# Autodesk Inventor part: finish
Saved by Autodesk Inventor 2022.2 (Build 262287000, 287)
## iProperties
Created: 2021-01-02
Part Number: finish
Material: Generic
Document SubType Name: Modeling
Designer: Tomasz
Density: 1 g/cm^3
Appearance: Default
Author: Tomasz
Autodesk Inventor part; units mm, degrees
ref_plane "YZ Plane" through (0, 0, 0) normal (1, 0, 0) x (0, 1, 0)
ref_plane "XZ Plane" through (0, 0, 0) normal (0, 1, 0) x (-1, 0, 0)
ref_plane "XY Plane" through (0, 0, 0) normal (0, 0, 1) x (1, 0, 0)
sketch "Sketch1" plane through (0, 0, 0) normal (0, 1, 0) x (-1, 0, 0)
  line L0 (275, 0) -> (-275, 0)
  line L1 (-275, 0) -> (-275, -720)
  line L2 (-275, -720) -> (275, -720)
  line L3 (275, -720) -> (275, 0)
  line L4 (255, 0) -> (255, -720)
  line L5 (-255, -720) -> (-255, 0)
  point P0 (0, 0)
  point P1 (0, 0)
  dimension "d0" = 550
  dimension "d1" = 720
  dimension "d4" = 20
  dimension "d5" = 20
  constraints: 12 end point, 4 point on line, 3 perpendicular, 2 parallel, 1 coincident, 1 horizontal, 1 midpoint
  measures "d0" distance of L2.end L1.end
  measures "d1" distance of L1.end L0.end
  measures "d4" distance between parallel lines of L1 L5
  measures "d5" distance between parallel lines of L3 L4
extrude "Extrusion1" add sketch "Sketch1" along normal blind 3
extrude "Extrusion2" add sketch "Sketch1" along normal blind 3.1 contours L3 L2 L4 L0 | L5 L2 L1 L0
sketch "Sketch2" plane through (0, 3, 0) normal (0, 1, 0) x (1, 0, 0)
  line L0 (-275, 0) -> (275, 0) projected
  line L1 (-275, 0) -> (-275, 550)
  line L2 (-275, 720) -> (-275, 0) projected
  line L3 (-275, 550) -> (-131, 550)
  line L4 (-131, 550) -> (-131, 540)
  line L5 (-131, 550) -> (-131, 560)
  line L6 (-131, 540) -> (-37, 540)
  line L7 (-131, 560) -> (-37, 560)
  line L8 (-37, 560) -> (-37, 540)
  line L9 (0, 0) -> (0, 720)
  line L10 (275, 550) -> (131, 550)
  line L11 (131, 550) -> (131, 540)
  line L12 (131, 550) -> (131, 560)
  line L13 (131, 540) -> (37, 540)
  line L14 (131, 560) -> (37, 560)
  line L15 (37, 560) -> (37, 540)
  dimension "d8" = 550
  dimension "d9" = 144
  dimension "d10" = 10
  dimension "d11" = 10
  dimension "d12" = 94
  constraints: 28 end point, 6 symmetric about line, 3 horizontal, 3 vertical, 1 perpendicular, 1 point on line
  measures "d8" distance of L0.start L1.end
  measures "d9" distance of L1.end L3.end
  measures "d10" distance of L3.end L4.end
  measures "d11" distance of L3.end L5.end
  measures "d12" distance of L4.end L6.end
sketch "Sketch4" plane through (0, 0, 0) normal (0, -1, 0) x (1, 0, 0)
  line L0 (-131, -540) -> (-37, -540) projected
  line L1 (131, -540) -> (37, -540) projected
  line L2 (37, -560) -> (37, -540) projected
  line L3 (131, -560) -> (37, -560) projected
  line L4 (131, -560) -> (131, -540)
  line L5 (131, -560) -> (37, -560)
  line L6 (37, -540) -> (131, -540)
  line L7 (37, -540) -> (37, -560)
  line L8 (-37, -540) -> (-37, -560)
  line L9 (-37, -560) -> (-131, -560)
  line L10 (-131, -560) -> (-131, -540)
  line L11 (-37, -540) -> (-131, -540)
  point P0 (0, 0)
  constraints: 16 end point, 5 equal length, 2 point on line, 1 perpendicular, 1 vertical
extrude "Extrusion5" cut sketch "Sketch2" against normal through all
extrude "Extrusion6" add sketch "Sketch4" against normal blind 3.1 separate body
equation "\"d0\" = track_width"
equation "\"d4\" = curb_width"
equation "\"d5\" = curb_width"
equation "\"d2\" = track_height"
equation "\"d6\" = track_height + curb_height"
equation "\"track_width\" = 550"
equation "\"curb_width\" = 20"
equation "\"track_height\" = 3"
equation "\"curb_height\" = 0.1"
body "Solid1"
body "Solid3"
